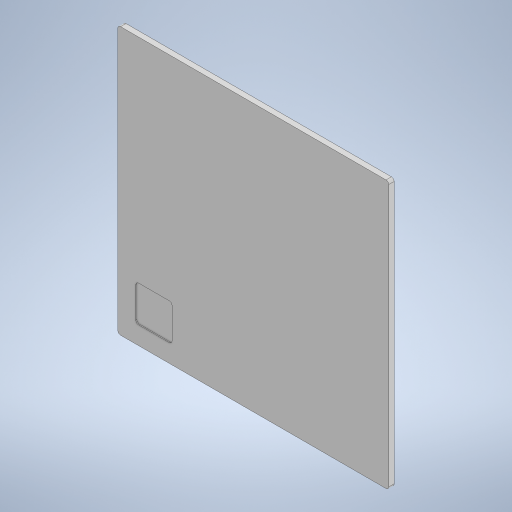
# Autodesk Inventor part: VacuumTableAdjustmentPlate
Saved by Autodesk Inventor 2024.2 (Build 282272000, 272)
## iProperties
Created: 2024-03-04
Part Number: VacuumTableAdjustmentPlate
Material: Generic
Document SubType Name: Modeling
Designer: lgnds
Density: 1 g/cm^3
Appearance: Default
Author: lgnds
Autodesk Inventor part; units mm, degrees
ref_plane "YZ Plane" through (0, 0, 0) normal (1, 0, 0) x (0, 1, 0)
ref_plane "XZ Plane" through (0, 0, 0) normal (0, 1, 0) x (-1, 0, 0)
ref_plane "XY Plane" through (0, 0, 0) normal (0, 0, 1) x (1, 0, 0)
sketch "Sketch1" plane through (0, 0, 0) normal (0, 0, 1) x (1, 0, 0)
  line L0 (-150, -148) -> (150, -148)
  line L1 (150, -148) -> (150, 148)
  line L2 (150, 148) -> (-150, 148)
  line L3 (-150, 148) -> (-150, -148)
  line L4 (-150, -148) -> (150, 148) construction
  line L5 (150, -148) -> (-150, 148) construction
  point P0 (0, 0)
  dimension "d0" = 296
  dimension "d1" = 300
  constraints: 12 end point, 2 midpoint, 2 parallel, 1 horizontal, 1 perpendicular
  measures "d0" distance between parallel lines of L0 L2
  measures "d1" distance between parallel lines of L1 L3
extrude "Extrusion1" add sketch "Sketch1" along normal blind 6
sketch "Sketch2" plane through (0, 0, 6) normal (0, 0, 1) x (1, 0, 0)
  line L0 (-130, -128) -> (-90, -128)
  line L1 (-90, -128) -> (-90, -88)
  line L2 (-90, -88) -> (-130, -88)
  line L3 (-130, -88) -> (-130, -128)
  line L4 (-150, 148) -> (-150, -148) projected
  line L5 (-150, -148) -> (150, -148) projected
  point P0 (0, 0)
  dimension "d4" = 20
  dimension "d5" = 20
  dimension "d6" = 40
  dimension "d7" = 40
  constraints: 8 end point, 2 parallel, 1 horizontal, 1 perpendicular
  measures "d4" distance between parallel lines of L4 L3
  measures "d5" distance between parallel lines of L5 L0
  measures "d6" distance between parallel lines of L0 L2
  measures "d7" distance between parallel lines of L3 L1
extrude "Extrusion2" cut sketch "Sketch2" against normal blind 1
fillet "Fillet1" radius 3 4 edges at (-130, -88, 5.5) (-90, -88, 5.5) (-90, -128, 5.5) (-130, -128, 5.5)
fillet "Fillet2" radius 3 4 edges at (-150, -148, 3) (150, -148, 3) (150, 148, 3) (-150, 148, 3)
equation "\"d5\" = d4"
body "Solid1"
